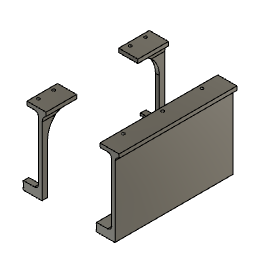
underCupboardShelveSupport v10 (Autodesk Fusion 360 design; units mm, degrees)
Autodesk Fusion 360 part; units mm, degrees
sketch "SideView" plane through (0, 0, 0) normal (0, 1, 0) x (1, 0, 0)
  line L0 (0, 0) -> (-20, 0)
  line L1 (-20, 0) -> (-20, -5)
  line L2 (-20, -5) -> (0, -5)
  line L3 (0, -5) -> (0, 0)
  line L4 (0, 0) -> (-5, 0)
  line L5 (-5, 0) -> (-5, 95)
  line L6 (-5, 95) -> (0, 95)
  line L7 (0, 95) -> (0, 0)
  line L8 (0, 95) -> (-24.5, 95)
  line L9 (-25, 95.5) -> (-25, 97.5)
  line L10 (-24.5, 98) -> (-0.5, 98)
  line L11 (0, 97.5) -> (0, 95)
  line L12 (-24.5, 87.2) -> (-5, 87.2)
  line L13 (-5, 87.2) -> (-5, 90.2)
  line L14 (-5, 90.2) -> (-24.5, 90.2)
  line L15 (-25, 89.7) -> (-25, 87.2)
  line L16 (-25, 98) -> (-25, 87.7) construction
  arc A0 (-25, 87.7) -> (-24.5, 87.2) centre (-24.5, 87.7) ccw
  arc A1 (-24.5, 90.2) -> (-25, 89.7) centre (-24.5, 89.7) ccw
  arc A2 (-25, 95.5) -> (-24.5, 95) centre (-24.5, 95.5) ccw
  arc A3 (-24.5, 98) -> (-25, 97.5) centre (-24.5, 97.5) ccw
  arc A4 (0, 97.5) -> (-0.5, 98) centre (-0.5, 97.5) ccw
  line L17 (0, -5) -> (5, -5)
  line L18 (5, -5) -> (5, 0)
  line L19 (5, 0) -> (0, 0)
  line L20 (0, 0) -> (0, -5)
  point P0 (-25, 95)
  dimension "d3" = 20
  dimension "d4" = 5
  dimension "d6" = 100
  dimension "d8" = 5
  dimension "d10" = 25
  dimension "d11" = 3
  dimension "d13" = 4.8
  dimension "d14" = 3
  dimension "d15" = 0.5
  dimension "d16" = 0.5
  dimension "d18" = 5
  constraint horizontal L0
  constraint vertical L1
  constraint horizontal L2
  constraint vertical L3
  constraint coincident L0.start L3.end
  constraint horizontal L4
  constraint vertical L5
  constraint horizontal L6
  constraint vertical L7
  constraint horizontal L8
  constraint vertical L9
  constraint horizontal L10
  constraint vertical L11
  constraint horizontal L12
  constraint vertical L13
  constraint horizontal L14
  constraint vertical L15
  constraint coincident L5 L13.end
  constraint perpendicular L8 L16
  constraint collinear L15 L16
  constraint coincident L15.end L12
  constraint tangent L12 A0
  constraint tangent L16 A0
  constraint tangent L14 A1
  constraint tangent L15 A1
  constraint equal A0 A1
  constraint coincident P0 L8
  constraint coincident P0 L9
  constraint tangent L8 A2
  constraint tangent L9 A2
  constraint equal A0 A2
  constraint coincident L16.start L9
  constraint coincident L16.start L10
  constraint tangent L9 A3
  constraint tangent L10 A3
  constraint equal A0 A3
  constraint tangent L11 A4
  constraint tangent L10 A4
  constraint horizontal L17
  constraint vertical L18
  constraint horizontal L19
  constraint vertical L20
  constraint equal L1 L20
  measures "d3" distance of L0.start L0.end
  measures "d4" distance of L0.start L2.end
  measures "d6" distance of L2.end L6.end
  measures "d8" distance of L5.end L6.end
  measures "d10" distance of L6.end P0
  measures "d11" distance of P0 L16.start
  measures "d13" distance of L8 L14
  measures "d14" distance of L12 L14
  measures "d15" radius of A0
  measures "d16" radius of A4
  measures "d18" distance of L3 L18
extrude "Extrude1" add sketch "SideView" along normal blind 154 makes body 1
fillet "Fillet1" radius 5 3 edges at (0, 77, 0) (-5, 77, 0) (-5, 77, -87.2) on bodies 1
fillet "Fillet2" radius 1.5 2 edges at (-5, 77, -90.2) (-5, 77, -95) on bodies 1
sketch "TopView" plane through (0, 0, 5) normal (0, 0, 1) x (-1, 0, 0)
  line L0 (20, 0) -> (-5, 0)
  line L1 (-5, 0) -> (-5, -154)
  line L2 (-5, -154) -> (20, -154)
  line L3 (20, -154) -> (20, 0)
  circle A0 centre (15, -25.6667) radius 1.8
  line L4 (15, 0) -> (15, -154) construction
  circle A1 centre (15, -128.3333) radius 1.8
  line L5 (15, -128.3333) -> (15, -25.6667)
  circle A2 centre (15, -77) radius 1.8
  point P0 (15, -77)
  dimension "d27" = 3.6
  dimension "d28" = 5
  dimension "d29" = 25.6667
  dimension "d31" = 3.6
  dimension "d32" = 25.6667
  dimension "d33" = 3.6
  constraint coincident L0 L4.start
  constraint coincident L2 L4.end
  constraint perpendicular L2 L4
  constraint coincident A0.centre L4
  constraint coincident L4 A1.centre
  constraint coincident A1.centre L5.start
  constraint coincident A0.centre L5.end
  constraint midpoint L4 P0
  constraint coincident P0 A2.centre
  measures "d27" diameter of A0
  measures "d28" distance of L2.end L4.end
  measures "d29" distance of L0 A0.centre
  measures "d31" diameter of A1
  measures "d32" distance of L2 A1.centre
  measures "d33" diameter of A2
extrude "Extrude2" cut sketch "TopView" against normal blind 5 contours A0 | A1 | L5 A2 | L5 A2 bodies 1
sketch "Sketch3" plane through (0, 0, 0) normal (0, 0, -1) x (1, 0, 0)
  line L0 (-10, -154) -> (-10, 0)
  line L1 (-10, 0) -> (-20, 0)
  line L2 (-20, 0) -> (-20, -154)
  line L3 (-20, -154) -> (-10, -154)
  circle A0 centre (-15, -25.6667) radius 3.5
  circle A1 centre (-15, -77) radius 3.5
  circle A2 centre (-15, -128.3333) radius 3.5
  circle A3 centre (-15, -128.3333) radius 1.8
  circle A4 centre (-15, -77) radius 1.8
  circle A5 centre (-15, -25.6667) radius 1.8
  point P0 (-15, -25.6667)
  point P1 (-15, -77)
  point P2 (-15, -128.3333)
  dimension "d36" = 7
  dimension "d37" = 7
  dimension "d38" = 7
  constraint concentric A0 A5
  constraint coincident P1 A1.centre
  constraint coincident P2 A2.centre
  measures "d36" diameter of A0
  measures "d37" diameter of A1
  measures "d38" diameter of A2
hole "Hole1" at (-15, 25.6667, 0) at (-15, 77, 0) at (-15, 128.3333, 0) direction (0, 0, 1) diameter 3.7 depth 10 tip angle 118 countersink diameter 7 countersink angle 90 bodies 1
sketch "Sketch4" plane through (0, 0, 0) normal (0, 1, 0) x (1, 0, 0)
  arc A0 (-5, 93.5) -> (-6.5, 95) centre (-6.5, 93.5) ccw
  line L0 (-5, 91.7) -> (-5, 93.5)
  arc A1 (-6.5, 90.2) -> (-5, 91.7) centre (-6.5, 91.7) ccw
  line L1 (-6.5, 90.2) -> (-24.5, 90.2)
  arc A2 (-5, 82.2) -> (-10, 87.2) centre (-10, 82.2) ccw
  line L2 (-5, 5) -> (-5, 82.2)
  arc A3 (-10, 0) -> (-5, 5) centre (-10, 5) ccw
  line L3 (-10, 0) -> (-20, 0)
  arc A4 (0, 5) -> (5, 0) centre (5, 5) ccw
  line L4 (0, 97.5) -> (0, 5)
  line L5 (-24.5, 87.2) -> (-10, 87.2)
  arc A5 (-25, 87.7) -> (-24.5, 87.2) centre (-24.5, 87.7) ccw
  line L6 (-25, 89.7) -> (-25, 87.7)
  arc A6 (-24.5, 90.2) -> (-25, 89.7) centre (-24.5, 89.7) ccw
  line L7 (-6.5, 95) -> (-24.5, 95)
  arc A7 (-25, 95.5) -> (-24.5, 95) centre (-24.5, 95.5) ccw
  line L8 (-25, 95.5) -> (-25, 97.5)
  arc A8 (-24.5, 98) -> (-25, 97.5) centre (-24.5, 97.5) ccw
  line L9 (-24.5, 98) -> (-0.5, 98)
  arc A9 (0, 97.5) -> (-0.5, 98) centre (-0.5, 97.5) ccw
  line L10 (5, -5) -> (5, 0)
  line L11 (-20, -5) -> (5, -5)
  line L12 (-20, 0) -> (-20, -5)
  line L13 (-24.5, 87.7) -> (-0.5, 87.7)
  line L14 (-0.5, 87.7) -> (-0.5, 97.5)
  line L15 (-0.5, 97.5) -> (-24.5, 97.5)
  line L16 (-24.5, 97.5) -> (-24.5, 87.7)
  constraint horizontal L13
  constraint vertical L14
  constraint horizontal L15
  constraint vertical L16
  constraint coincident A9.centre L14.end
  constraint coincident A5.centre L13.start
extrude "Extrude3" add sketch "Sketch4" along normal blind 1 contours A0 L0 A1 L1 L7 L16 | A0 L0 A1 L1 L7 L13 L14 L15 L16 bodies 1
sketch "Sketch5" plane through (0, 154, 0) normal (0, 1, 0) x (-1, 0, 0)
  line L0 (10, 0) -> (20, 0)
  line L1 (20, 0) -> (20, 5)
  line L2 (20, 5) -> (-5, 5)
  line L3 (-5, 5) -> (-5, 0)
  arc A0 (0, -5) -> (-5, 0) centre (-5, -5) ccw
  line L4 (0, -5) -> (0, -97.5)
  arc A1 (0, -97.5) -> (0.5, -98) centre (0.5, -97.5) ccw
  line L5 (0.5, -98) -> (24.5, -98)
  arc A2 (24.5, -98) -> (25, -97.5) centre (24.5, -97.5) ccw
  line L6 (25, -97.5) -> (25, -95.5)
  arc A3 (25, -95.5) -> (24.5, -95) centre (24.5, -95.5) ccw
  line L7 (24.5, -95) -> (6.5, -95)
  arc A4 (5, -93.5) -> (6.5, -95) centre (6.5, -93.5) ccw
  line L8 (5, -93.5) -> (5, -91.7)
  arc A5 (6.5, -90.2) -> (5, -91.7) centre (6.5, -91.7) ccw
  line L9 (6.5, -90.2) -> (24.5, -90.2)
  arc A6 (24.5, -90.2) -> (25, -89.7) centre (24.5, -89.7) ccw
  line L10 (25, -89.7) -> (25, -87.7)
  arc A7 (25, -87.7) -> (24.5, -87.2) centre (24.5, -87.7) ccw
  line L11 (24.5, -87.2) -> (10, -87.2)
  arc A8 (5, -82.2) -> (10, -87.2) centre (10, -82.2) ccw
  line L12 (5, -82.2) -> (5, -5)
  arc A9 (10, 0) -> (5, -5) centre (10, -5) ccw
  line L13 (24.5, -95) -> (24.5, -90.2)
  arc A10 (25, -95.5) -> (24.5, -95) centre (24.5, -95.5) ccw
  line L14 (25, -95.5) -> (25, -97.5)
  arc A11 (24.5, -98) -> (25, -97.5) centre (24.5, -97.5) ccw
  line L15 (24.5, -98) -> (0.5, -98)
  arc A12 (0, -97.5) -> (0.5, -98) centre (0.5, -97.5) ccw
  line L16 (0, -97.5) -> (0, -5)
  arc A13 (0, -5) -> (-5, 0) centre (-5, -5) ccw
  line L17 (-5, 5) -> (-5, 0)
  line L18 (20, 5) -> (-5, 5)
  line L19 (20, 0) -> (20, 5)
  line L20 (10, 0) -> (20, 0)
  arc A14 (10, 0) -> (5, -5) centre (10, -5) ccw
  line L21 (5, -5) -> (5, -82.2)
  arc A15 (5, -82.2) -> (10, -87.2) centre (10, -82.2) ccw
  line L22 (24.5, -87.2) -> (10, -87.2)
  arc A16 (25, -87.7) -> (24.5, -87.2) centre (24.5, -87.7) ccw
  line L23 (25, -89.7) -> (25, -87.7)
  arc A17 (24.5, -90.2) -> (25, -89.7) centre (24.5, -89.7) ccw
  line L24 (24.5, -87.7) -> (0.5, -87.7)
  line L25 (0.5, -87.7) -> (0.5, -97.5)
  line L26 (0.5, -97.5) -> (24.5, -97.5)
  line L27 (24.5, -97.5) -> (24.5, -87.7)
  constraint horizontal L24
  constraint vertical L25
  constraint horizontal L26
  constraint vertical L27
  constraint coincident A1.centre A12.centre
  constraint coincident A7.centre A16.centre
extrude "Extrude4" add sketch "Sketch5" against normal blind 1 contours L7 A4 L8 A5 L9 L13 L27 | L7 A4 L8 A5 L9 L24 L25 L26 L27 bodies 1
fillet "Fillet4" radius 1 5 edges at (-15.5, 153, -90.2) (-5.4393, 153, -90.6393) (-5, 153, -92.6) (-5.4393, 153, -94.5607) (-15.5, 153, -95) on bodies 1
fillet "Fillet5" radius 1 5 edges at (-15.5, 1, -95) (-5.4393, 1, -94.5607) (-5, 1, -92.6) (-5.4393, 1, -90.6393) (-15.5, 1, -90.2) on bodies 1
sketch "Sketch1" plane through (0, 0, 0) normal (0, 1, 0) x (1, 0, 0) in component "SmallerLeft"
  line L0 (-95.4651, 0.408) -> (-115.4651, 0.408)
  line L1 (-120.4651, 98.408) -> (-120.4651, 88.108) construction
  line L2 (-95.4651, -4.592) -> (-90.4651, -4.592)
  line L3 (-90.4651, -4.592) -> (-90.4651, 0.408)
  line L4 (-90.4651, 0.408) -> (-95.4651, 0.408)
  arc A0 (-120.4651, 95.908) -> (-119.9651, 95.408) centre (-119.9651, 95.908) ccw
  arc A1 (-119.9651, 90.608) -> (-120.4651, 90.108) centre (-119.9651, 90.108) ccw
  line L5 (-95.4651, -4.592) -> (-95.4651, 0.408)
  line L6 (-95.4651, 95.408) -> (-95.4651, 0.408)
  line L7 (-120.4651, 95.908) -> (-120.4651, 97.908)
  line L8 (-119.9651, 87.608) -> (-100.4651, 87.608)
  line L9 (-100.4651, 87.608) -> (-100.4651, 90.608)
  line L10 (-120.4651, 90.108) -> (-120.4651, 87.608)
  line L11 (-100.4651, 90.608) -> (-119.9651, 90.608)
  arc A2 (-95.4651, 97.908) -> (-95.9651, 98.408) centre (-95.9651, 97.908) ccw
  arc A3 (-120.4651, 88.108) -> (-119.9651, 87.608) centre (-119.9651, 88.108) ccw
  line L12 (-119.9651, 98.408) -> (-95.9651, 98.408)
  line L13 (-95.4651, 95.408) -> (-119.9651, 95.408)
  line L14 (-115.4651, 0.408) -> (-115.4651, -4.592)
  arc A4 (-119.9651, 98.408) -> (-120.4651, 97.908) centre (-119.9651, 97.908) ccw
  line L15 (-100.4651, 0.408) -> (-100.4651, 95.408)
  line L16 (-115.4651, -4.592) -> (-95.4651, -4.592)
  line L17 (-100.4651, 95.408) -> (-95.4651, 95.408)
  line L18 (-95.4651, 0.408) -> (-95.4651, -4.592)
  line L19 (-95.4651, 97.908) -> (-95.4651, 95.408)
  line L20 (-95.4651, 0.408) -> (-100.4651, 0.408)
  line L21 (-119.9651, 90.108) -> (-95.9651, 90.108)
  line L22 (-95.9651, 90.108) -> (-95.9651, 98.408)
  line L23 (-95.9651, 98.408) -> (-119.9651, 98.408)
  line L24 (-119.9651, 98.408) -> (-119.9651, 90.108)
  point P0 (-120.4651, 95.408)
  point P1 (-95.4651, 0.408)
  dimension "d54" = 20
  dimension "d55" = 5
  dimension "d56" = 100
  dimension "d57" = 5
  dimension "d58" = 25
  dimension "d59" = 3
  dimension "d60" = 4.8
  dimension "d61" = 3
  dimension "d62" = 0.5
  dimension "d63" = 0.5
  dimension "d64" = 5
  constraint horizontal L0
  constraint vertical L14
  constraint horizontal L16
  constraint vertical L5
  constraint coincident P1 L0.start
  constraint horizontal L20
  constraint vertical L15
  constraint horizontal L17
  constraint vertical L6
  constraint horizontal L13
  constraint vertical L7
  constraint horizontal L12
  constraint vertical L19
  constraint horizontal L8
  constraint vertical L9
  constraint horizontal L11
  constraint vertical L10
  constraint coincident L9.end L15
  constraint perpendicular L1 L13
  constraint collinear L1 L10
  constraint coincident L10.end L8
  constraint tangent L8 A3
  constraint tangent L1 A3
  constraint tangent A1 L11
  constraint tangent A1 L10
  constraint equal A1 A3
  constraint coincident P0 L13
  constraint coincident P0 L7
  constraint tangent A0 L13
  constraint tangent A0 L7
  constraint equal A0 A3
  constraint coincident L1.start L7
  constraint coincident L1.start L12
  constraint tangent L7 A4
  constraint tangent L12 A4
  constraint equal A3 A4
  constraint tangent A2 L19
  constraint tangent A2 L12
  constraint horizontal L2
  constraint vertical L3
  constraint horizontal L4
  constraint vertical L18
  constraint equal L14 L18
  constraint horizontal L21
  constraint vertical L22
  constraint horizontal L23
  constraint vertical L24
  constraint coincident A1.centre L21.start
  measures "d54" distance of L0.end P1
  measures "d55" distance of L2.start P1
  measures "d56" distance of L6.start L2.start
  measures "d57" distance of L6.start L15.end
  measures "d58" distance of P0 L6.start
  measures "d59" distance of P0 L1.start
  measures "d60" distance of L11 L13
  measures "d61" distance of L8 L11
  measures "d62" radius of A3
  measures "d63" radius of A2
  measures "d64" distance of L3 L5
extrude "Extrude1'" add sketch "Sketch1" along normal blind 40 separate body contours L0 L5 L14 L16 L18 L20 | L2 L3 L4 L5 L18 | L0 L6 L9 L13 L15 L17 L20 L21 L22 | A2 L13 L17 L19 L22 | A1 L8 L9 L10 A3 L15 L21 L24 | L9 L13 L15 L17 L21 L22 | L12 L13 L17 L22 L23 L24 | L9 L11 L15 L21 L24 | A0 L7 A4 L24 makes body 2 in component "SmallerLeft"
extrude "Extrude2'" add sketch "Sketch1" along normal blind 1 contours L11 L13 L15 L24 bodies 2 in component "SmallerLeft"
sketch "Sketch2" plane through (0, 0, 4.592) normal (0, 0, 1) x (-1, 0, 0) in component "SmallerLeft"
  line L0 (115.4651, 0) -> (90.4651, 0)
  line L1 (90.4651, 0) -> (90.4651, -40)
  line L2 (90.4651, -40) -> (115.4651, -40)
  line L3 (115.4651, -40) -> (115.4651, 0)
  line L4 (110.4651, -40) -> (110.4651, 0) construction
  line L5 (110.4651, -20) -> (90.4651, -20) construction
  point P0 (110.4651, -20)
  point P1 (110.4651, -30)
  dimension "d70" = 5
  dimension "d71" = 10
  constraint coincident L2 L4.start
  constraint coincident L0 L4.end
  constraint perpendicular L0 L4
  constraint midpoint L4 P0
  constraint coincident P0 L5.start
  constraint midpoint L1 L5.end
  constraint coincident L4 P1
  measures "d70" distance of L3 L4
  measures "d71" distance of L4.start P1
sketch "Sketch3 (2)" plane through (0, 0, -0.408) normal (0, 0, -1) x (1, 0, 0) in component "SmallerLeft"
  line L0 (-100.4651, 0) -> (-115.4651, 0)
  line L1 (-115.4651, 0) -> (-115.4651, -40)
  line L2 (-115.4651, -40) -> (-100.4651, -40)
  line L3 (-100.4651, -40) -> (-100.4651, 0)
  line L4 (-110.4651, -40) -> (-110.4651, 0)
  line L5 (-110.4651, -20) -> (-90.4651, -20)
  line L6 (-110.4651, -20) -> (-90.4651, -20) construction
  point P0 (-110.4651, -20)
  point P1 (-110.4651, -30)
  point P2 (-110.4651, -40)
  point P3 (-110.4651, -10)
  constraint coincident P0 L5.start
  constraint coincident L5.end L6.end
  constraint symmetric P1 L6 P3
hole "Hole1'" at (-110.4651, 30, -0.408) direction (0, 0, 1) diameter 3.6 depth 7 tip angle 118 countersink diameter 7 countersink angle 90 bodies 2 in component "SmallerLeft"
hole "Hole2" at (-110.4651, 10, -0.408) direction (0, 0, 1) diameter 3.6 depth 7 tip angle 118 countersink diameter 7 countersink angle 90 bodies 2 in component "SmallerLeft"
sketch "Sketch4 (2)" plane through (-95.4651, 0, 0) normal (1, 0, 0) x (0, 1, 0) in component "SmallerLeft"
  line L0 (0, -0.408) -> (0, -97.908)
  line L1 (0, -97.908) -> (40, -97.908)
  line L2 (40, -97.908) -> (40, -0.408)
  line L3 (40, -0.408) -> (0, -0.408)
  line L4 (0, -95.408) -> (0, -90.608)
  line L5 (0, 4.592) -> (40, 4.592)
  line L6 (0, -0.408) -> (0, 4.592)
  line L7 (40, -0.408) -> (40, 4.592)
  line L8 (0, -0.408) -> (0, -87.608)
  line L9 (40, -87.608) -> (40, -0.408)
  line L10 (0, -88.108) -> (0, -87.608)
  line L11 (40, -88.108) -> (40, -87.608)
  line L12 (0, -90.108) -> (0, -88.108)
  line L13 (40, -90.108) -> (40, -88.108)
  line L14 (0, -90.608) -> (0, -90.108)
  line L15 (40, -90.608) -> (40, -90.108)
  line L16 (40, -95.408) -> (40, -90.608)
  line L17 (0, -95.908) -> (0, -95.408)
  line L18 (40, -95.908) -> (40, -95.408)
  line L19 (0, -95.908) -> (0, -97.908)
  line L20 (40, -97.908) -> (40, -95.908)
  line L21 (0, -98.408) -> (0, -97.908)
  line L22 (40, -98.408) -> (40, -97.908)
  line L23 (0, -98.408) -> (40, -98.408)
  line L24 (0, 4.592) -> (0, -98.408)
  line L25 (0, -98.408) -> (7, -98.408)
  line L26 (7, -98.408) -> (7, -32.908)
  line L27 (40, -0.408) -> (39.5, -0.408)
  arc A0 (39.5, -0.408) -> (7, -32.908) centre (39.5, -32.908) ccw
  line L28 (40, -0.408) -> (40, -98.408)
  line L29 (40, -98.408) -> (0, -98.408)
  dimension "d83" = 7
  dimension "d84" = 32.5
  constraint coincident L5.start L6.end
  constraint coincident L21.start L23.start
  constraint perpendicular L24 L25
  constraint perpendicular L5 L26
  constraint coincident L2.end L3.start
  constraint tangent L27 A0
  constraint tangent L26 A0
  constraint coincident L22.start L23.end
  measures "d83" distance of L21.start L25.end
  measures "d84" radius of A0
extrude "Extrude3'" cut sketch "Sketch4 (2)" against normal blind 25 contours L1 L2 L3 L9 L11 L13 L15 L16 L18 L20 L26 L27 A0 L28 | L1 L22 L23 L26 L28 L29 bodies 2 in component "SmallerLeft"
fillet "Fillet1'" radius 10 1 edges at (-95.4651, 19.75, -0.408) on bodies 2 in component "SmallerLeft"
fillet "Fillet2'" radius 5 1 edges at (-100.4651, 19.75, -0.408) on bodies 2 in component "SmallerLeft"
ref_plane "WorkPlane2" through (-102.9651, 80, 2.092) normal (0, 1, 0) x (1, 0, 0) in component "SmallerLeft"
mirror "Mirror1" about plane through (-102.9651, 80, 2.092) normal (0, 1, 0) of bodies 2 makes body 3 in component "SmallerLeft"
fillet "Fillet4'" radius 1.5 4 edges at (-100.4651, 4, -90.608) (-100.4651, 4, -95.408) (-100.4651, 156, -90.608) (-100.4651, 156, -95.408) on bodies 2 3 in component "SmallerLeft"
fillet "Fillet5'" radius 0.6 10 edges at (-110.9651, 1, -95.408) (-100.9045, 1, -94.9686) (-100.4651, 1, -93.008) (-100.9045, 1, -91.0473) (-110.9651, 1, -90.608) (-110.9651, 159, -95.408) (-100.9045, 159, -94.9686) (-100.4651, 159, -93.008) (-100.9045, 159, -91.0473) (-110.9651, 159, -90.608) on bodies 2 3 in component "SmallerLeft"
fillet "Fillet6" radius 5 2 edges at (-100.4651, 3.5, -87.608) (-100.4651, 156.5, -87.608) on bodies 2 3 in component "SmallerLeft"
component "SmallerLeft" placed x (1, 0, 0) y (0, 1, 0) z (0, 0, 1) at (0, 0, 0)
equation "BaseWidth = 18 mm"
equation "ScrewLength = 20 mm"
equation "d4 = ScrewLength - BaseWidth + 3 mm"
equation "HangeDepth = 100 mm"
equation "d6 = HangeDepth"
equation "SupportWidth = 5 mm"
equation "d8 = SupportWidth"
equation "ShelfClipWidth = 3 mm"
equation "d11 = ShelfClipWidth"
equation "ShelveWidth = 4.8 mm"
equation "d13 = ShelveWidth"
equation "d14 = ShelfClipWidth"
equation "ShelfDelth = 154 mm"
equation "d18 = SupportWidth"
equation "d19 = ShelfDelth"
equation "ScrewHead = 7 mm"
equation "ScrewBody = 3.6 mm"
equation "d27 = ScrewBody"
equation "d29 = ShelfDelth / 6"
equation "d31 = ScrewBody"
equation "d32 = ShelfDelth / 6"
equation "d33 = ScrewBody"
equation "d34 = -( ScrewLength - BaseWidth + 3 mm )"
equation "d36 = ScrewHead"
equation "d37 = ScrewHead"
equation "d38 = ScrewHead"
equation "d55 = ScrewLength - BaseWidth + 3 mm"
equation "d56 = HangeDepth"
equation "d57 = SupportWidth"
equation "d59 = ShelfClipWidth"
equation "d60 = ShelveWidth"
equation "d61 = ShelfClipWidth"
equation "d64 = SupportWidth"
equation "LeftBaseDepth = 40 mm"
equation "d66 = LeftBaseDepth"
equation "d73 = ScrewBody"
equation "d75 = ScrewHead"
equation "d78 = ScrewBody"
equation "d80 = ScrewHead"
equation "LeftBaseThinDepth = 7 mm"
equation "d83 = LeftBaseThinDepth"
named bodies: "ShelfSupport", "LeftShelfBracket", "RightShelfBracket"
